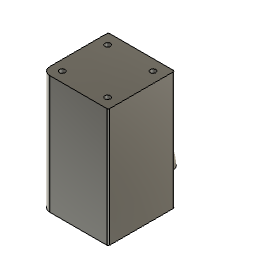
Leg_Extension_Front_Right (Autodesk Fusion 360 design; units mm, degrees)
Autodesk Fusion 360 part; units mm, degrees
sketch "Skizze1" plane through (0, 0, 0) normal (0, 0, 1) x (1, 0, 0)
  line L0 (0, 0) -> (50.5, 0)
  line L1 (50.5, 0) -> (50.5, 50.5)
  line L2 (50.5, 50.5) -> (0, 50.5)
  line L3 (0, 50.5) -> (0, 0)
  line L4 (0, 50.5) -> (20.1, 50.5)
  line L5 (20.1, 50.5) -> (20.1, 80.5)
  line L6 (20.1, 50.5) -> (25.1, 50.5)
  line L7 (25.1, 50.5) -> (25.1, 75.5)
  line L8 (20.1, 80.5) -> (25.1, 75.5)
  line L9 (50.5, 0) -> (50.5, 20.1)
  line L10 (50.5, 20.1) -> (50.5, 25.1)
  circle A0 centre (25, 25) radius 12.7
  line L11 (42.25, 42.25) -> (7.75, 42.25)
  line L12 (7.75, 42.25) -> (7.75, 7.75)
  line L13 (7.75, 7.75) -> (42.25, 7.75)
  line L14 (42.25, 7.75) -> (42.25, 42.25)
  line L15 (42.25, 42.25) -> (7.75, 7.75) construction
  line L16 (7.75, 42.25) -> (42.25, 7.75) construction
  point P0 (25, 25)
  dimension "d1" = 50.5
  dimension "d2" = 50.5
  dimension "d3" = 20.1
  dimension "d4" = 30
  dimension "d5" = 5
  dimension "d6" = 25
  dimension "d13" = 25.4
  dimension "d14" = 34.5
  dimension "d15" = 34.5
  constraint horizontal L0
  constraint horizontal L2
  constraint vertical L3
  constraint coincident L0.start L3.end
  constraint perpendicular L3 L4
  constraint perpendicular L4 L5
  constraint perpendicular L5 L6
  constraint perpendicular L6 L7
  constraint perpendicular L0 L9
  constraint perpendicular L11 L12
  constraint parallel L11 L13
  constraint parallel L12 L14
  constraint horizontal L11
  constraint coincident L15 P0
  constraint coincident L16 P0
  constraint coincident P0 A0.centre
  measures "d1" distance of L0.start L0.end
  measures "d2" distance of L0.start L2.end
  measures "d3" distance of L2.end L4.end
  measures "d4" distance of L4.end L5.end
  measures "d5" distance of L4.end L6.end
  measures "d6" distance of L6.end L7.end
  measures "d13" diameter of A0
  measures "d14" distance of L12.end L13.end
  measures "d15" distance of L11.end L12.end
extrude "Extrusion1" add sketch "Skizze1" along normal blind 90 contours L0 L1 L2 L3 L4 L6 L9 L10 | A0 | L11 L12 L13 L14
extrude "Extrusion2" cut sketch "Skizze1" along normal blind 15 contours A0
chamfer "Fase1" distance 2.5 distance2 15 1 edges at (13.1594, 20.4075, 0) measured on face at (25.483, 46.2215, 0)
sketch "Skizze2" plane through (0, 0, 0) normal (0, 0, -1) x (1, 0, 0)
  line L0 (0, 0) -> (0, -50.5)
  line L1 (0, -50.5) -> (50.5, -50.5)
  line L2 (50.5, -50.5) -> (50.5, 0)
  line L3 (50.5, 0) -> (0, 0)
  circle A0 centre (25, -25) radius 15.2
  line L4 (42.25, -7.75) -> (7.75, -7.75)
  line L5 (7.75, -7.75) -> (7.75, -42.25)
  line L6 (7.75, -42.25) -> (42.25, -42.25)
  line L7 (42.25, -42.25) -> (42.25, -7.75)
  line L8 (42.25, -7.75) -> (7.75, -42.25) construction
  line L9 (7.75, -7.75) -> (42.25, -42.25) construction
  point P0 (25, -25)
  dimension "d20" = 34.5
  dimension "d21" = 34.5
  constraint perpendicular L4 L5
  constraint parallel L4 L6
  constraint parallel L5 L7
  constraint horizontal L4
  constraint coincident L8 P0
  constraint coincident L9 P0
  constraint coincident P0 A0.centre
  measures "d20" distance of L5.end L6.end
  measures "d21" distance of L4.end L5.end
hole "Bohrung1" at (42.25, 7.75, 0) at (7.75, 7.75, 0) at (7.75, 42.25, 0) at (42.25, 42.25, 0) direction (0, 0, 1) diameter 8.8 depth 82 tip angle 180
hole "Bohrung2" at (7.75, 7.75, 82) direction (0, 0, 1) diameter 4.2 depth 82 tip angle 180 countersink diameter 8.6 countersink angle 90
hole "Bohrung3" at (42.25, 7.75, 82) direction (0, 0, 1) diameter 4.2 depth 82 tip angle 180 countersink diameter 8.6 countersink angle 90
hole "Bohrung4" at (42.25, 42.25, 82) direction (0, 0, 1) diameter 4.2 depth 82 tip angle 180 countersink diameter 8.6 countersink angle 90
hole "Bohrung5" at (7.75, 42.25, 82) direction (0, 0, 1) diameter 4.2 depth 82 tip angle 180 countersink diameter 8.6 countersink angle 90
ref_plane "Arbeitsebene2" through (20.1, 65.5, 0) normal (1, 0, 0) x (0, 1, 0)
sketch "Skizze4" plane through (20.1, 65.5, 0) normal (1, 0, 0) x (0, 1, 0)
  line L0 (-15, 0) -> (15, 0)
  line L1 (-15, 0) -> (-15, 30)
  arc A0 (15, 0) -> (-15, 30) centre (-15, 0) ccw
  dimension "d52" = 30
  dimension "d53" = 30
  constraint horizontal L0
  constraint perpendicular L0 L1
  measures "d52" distance of L0.start L0.end
  measures "d53" distance of L0.start L1.end
extrude "Extrusion4" add sketch "Skizze4" along normal blind 5
fillet "Fillet5" radius 6 1 edges at (0, 0, 45)
fillet "Fillet6" radius 1 3 edges at (0, 50.5, 45) (50.5, 0, 45) (50.5, 50.5, 45)
fillet "Fillet7" radius 6 1 edges at (25.1, 71.7132, 21.2132)
